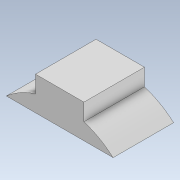
# Autodesk Inventor part: Capston_Disc_Flachstelle
Saved by Autodesk Inventor 2022 (Build 260153000, 153)
## iProperties
Created: 2022-09-13
Part Number: Capston_Disc_Flachstelle
Material: Generisch
Document SubType Name: Modeling
Designer: alexw
Density: 1 g/cm^3
Appearance: Vorgabe
Wellennuttiefe_40: 5,000 mm
Nabennuttiefe_40: 3,300 mm
D: 40,000 mm
Author: alexw
Autodesk Inventor part; units mm, degrees
ref_plane "YZ Plane" through (0, 0, 0) normal (1, 0, 0) x (0, 1, 0)
ref_plane "XZ Plane" through (0, 0, 0) normal (0, 1, 0) x (-1, 0, 0)
ref_plane "XY Plane" through (0, 0, 0) normal (0, 0, 1) x (1, 0, 0)
sketch "Skizze1" plane through (0, 0, 0) normal (0, 0, 1) x (1, 0, 0)
  line L0 (-6, 8.3) -> (6, 8.3)
  line L1 (0, 0) -> (0, 8.3) construction
  line L2 (-6, 8.3) -> (-6, 4.0788)
  circle A0 centre (0, -15) radius 20 construction
  line L3 (6, 8.3) -> (6, 4.0788)
  line L4 (-6, 4.0788) -> (6, 4.0788) construction
  line L5 (-13.2288, 0) -> (13.2288, 0)
  arc A1 (-6, 4.0788) -> (-13.2288, 0) centre (0, -15) ccw
  arc A2 (13.2288, 0) -> (6, 4.0788) centre (0, -15) ccw
  point P0 (0, 5)
  dimension "d0" = 40
  dimension "d1" = 12
  dimension "d2" = 3.3
  dimension "d3" = 5
  constraints: 12 end point, 9 point on circle, 3 centre point, 3 horizontal, 3 vertical, 2 concentric, 2 midpoint, 1 parallel, 1 point on line
  measures "d0" diameter of A0
  measures "d1" distance between parallel lines of L3 L2
  measures "d2" distance from line of L0 point (0, 5)
  measures "d3" distance from line of L5 point (0, 5)
extrude "Extrusion1" add sketch "Skizze1" along normal blind 15
equation "\"d0\" = D"
equation "\"d1\" = Passfeder_Width_40"
equation "\"d2\" = Nabennuttiefe_40"
equation "\"d3\" = Wellennuttiefe_40"
equation "\"D\" = 40"
equation "\"Passfeder_Width_40\" = 12"
equation "\"Nabennuttiefe_40\" = 3.3"
equation "\"Wellennuttiefe_40\" = 5"
